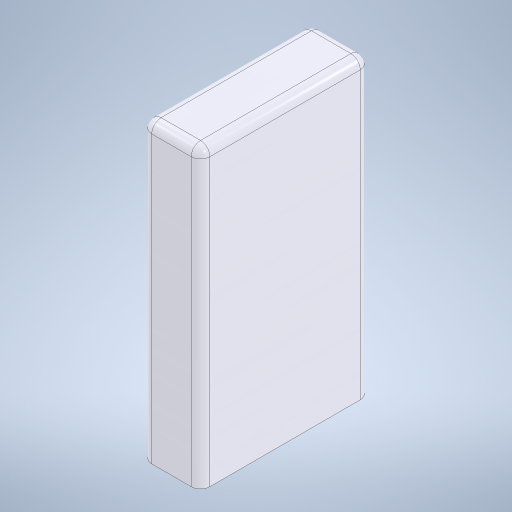
# Autodesk Inventor part: batt
Saved by Autodesk Inventor 2024.1 (Build 281209000, 209)
## iProperties
Created: 2024-04-29
Part Number: batt
Material: Générique
Document SubType Name: Modeling
Designer: chass
Density: 1 g/cm^3
Appearance: Par défaut
Author: chass
Autodesk Inventor part; units mm, degrees
ref_plane "YZ Plane" through (0, 0, 0) normal (1, 0, 0) x (0, 1, 0)
ref_plane "XZ Plane" through (0, 0, 0) normal (0, 1, 0) x (-1, 0, 0)
ref_plane "XY Plane" through (0, 0, 0) normal (0, 0, 1) x (1, 0, 0)
sketch "Esquisse1" plane through (0, 0, 0) normal (0, 1, 0) x (-1, 0, 0)
  line L0 (10, 69) -> (-21, 69)
  line L1 (-21, 69) -> (-21, -21)
  line L2 (-21, -21) -> (10, -21)
  line L3 (10, -21) -> (10, 69)
  point P0 (0, 0)
  dimension "d0" = 90
  dimension "d1" = 31
  constraints: 8 end point, 2 parallel, 1 horizontal, 1 perpendicular
  measures "d0" distance of L2.end L0.start
  measures "d1" distance of L1.end L2.end
extrude "Extrusion1" add sketch "Esquisse1" along normal blind 157
fillet "Congé1" radius 5 8 edges at (21, 157, 24) (-10, 157, 24) (5.5, 157, 69) (5.5, 157, -21) (21, 78.5, -21) (-10, 78.5, -21) (-10, 78.5, 69) (21, 78.5, 69)
